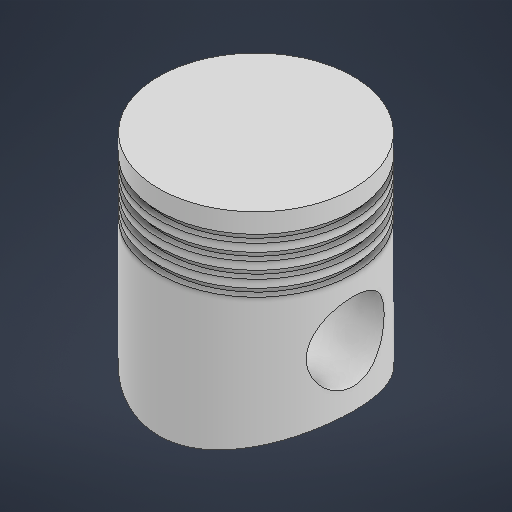
# Autodesk Inventor part: piston
Saved by Autodesk Inventor 2026.1 (Build 301233020, 233B)
## iProperties
Created: 2025-12-09
Part Number: piston
Material: Generic
Document SubType Name: Modeling
Designer: ender
Mass: 105.48 g
Surface Area: 374.417 cm^2
Volume: 105.48 cm^3
Density: 1 g/cm^3
Appearance: Default
Author: ender
Autodesk Inventor part; units mm, degrees
ref_plane "YZ Plane" through (0, 0, 0) normal (1, 0, 0) x (0, 1, 0)
ref_plane "XZ Plane" through (0, 0, 0) normal (0, 1, 0) x (-1, 0, 0)
ref_plane "XY Plane" through (0, 0, 0) normal (0, 0, 1) x (1, 0, 0)
sketch "Sketch1" plane through (0, 0, 0) normal (0, 0, 1) x (1, 0, 0)
  line L0 (0, 0) -> (31.75, 0)
  line L1 (31.75, 0) -> (31.75, -5.08)
  line L2 (31.75, -5.08) -> (0, -5.08)
  line L3 (0, -5.08) -> (0, 0)
  line L4 (31.75, -5.08) -> (26.67, -5.08)
  line L5 (26.67, -5.08) -> (26.67, -69.85)
  line L6 (26.67, -69.85) -> (31.75, -69.85)
  line L7 (31.75, -69.85) -> (31.75, -5.08)
  line L8 (0, 0) -> (0, 62.0882)
  line L9 (31.75, -6.35) -> (29.718, -6.35)
  line L10 (29.718, -6.35) -> (29.718, -8.89)
  line L11 (29.718, -8.89) -> (31.75, -8.89)
  line L12 (31.75, -8.89) -> (31.75, -6.35)
  line L13 (31.75, -11.43) -> (29.718, -11.43)
  line L14 (29.718, -11.43) -> (29.718, -13.97)
  line L15 (29.718, -13.97) -> (31.75, -13.97)
  line L16 (31.75, -13.97) -> (31.75, -11.43)
  line L17 (31.75, -16.51) -> (29.718, -16.51)
  line L18 (29.718, -16.51) -> (29.718, -19.05)
  line L19 (29.718, -19.05) -> (31.75, -19.05)
  line L20 (31.75, -19.05) -> (31.75, -16.51)
  line L21 (31.75, -21.59) -> (29.718, -21.59)
  line L22 (29.718, -21.59) -> (29.718, -24.13)
  line L23 (29.718, -24.13) -> (31.75, -24.13)
  line L24 (31.75, -24.13) -> (31.75, -21.59)
  line L25 (0, -96.2376) -> (0, 88.4758) projected
  dimension "d0" = 69.85
  dimension "d1" = 5.08
  dimension "d2" = 63.5
  dimension "d3" = 2.032
  dimension "d4" = 2.54
  dimension "d5" = 6.35
  dimension "d6" = 5.08
  dimension "d7" = 5.08
  dimension "d8" = 5.08
  constraints: 50 end point, 12 parallel, 6 horizontal, 6 perpendicular, 6 point on line, 4 equal length, 1 collinear, 1 vertical
  measures "d0" distance between parallel lines of L6 L0
  measures "d1" distance of L5.end L6.end
  measures "d2" diameter of L1 L8
  measures "d3" distance of L9.start L9.end
  measures "d4" distance of L9.end L10.end
  measures "d5" distance between parallel lines of L9 L0
  measures "d6" distance between parallel lines of L15 L11
  measures "d7" distance between parallel lines of L19 L15
  measures "d8" distance between parallel lines of L23 L19
revolve "Revolution1" add sketch "Sketch1" angle 360 about axis through (0, -10, 0) along (0, 1, 0) contours L0 L1 L2 L3 | L7 L9 L10 L11 L13 L14 L15 L17 L18 L19 L21 L22 L23 L6 L5 L2
sketch "Sketch2" plane through (0, -5.08, 0) normal (0, -1, 0) x (1, 0, 0)
  circle A0 centre (0, 0) radius 26.67 projected
  line L0 (20.9454, 16.51) -> (10.16, 16.51)
  line L1 (10.16, 16.51) -> (10.16, -16.51)
  line L2 (10.16, -16.51) -> (20.9454, -16.51)
  line L3 (-20.9454, 16.51) -> (-10.16, 16.51)
  line L4 (-10.16, 16.51) -> (-10.16, -16.51)
  line L5 (-10.16, -16.51) -> (-20.9454, -16.51)
  dimension "d10" = 33.02
  dimension "d11" = 20.32
  constraints: 12 end point, 4 equal length, 4 perpendicular, 4 point on circle, 2 horizontal
  measures "d10" distance between parallel lines of L5 L3
  measures "d11" distance between parallel lines of L4 L1
extrude "Extrusion1" add sketch "Sketch2" along normal blind 55.88 contours A0 L2 L1 L0 | L3 L4 L5 A0
sketch "Sketch3" plane through (-10.16, -5.08, 16.51) normal (1, 0, 0) x (0, 0, -1)
  circle A0 centre (16.51, -38.1) radius 12.7
  line L0 (48.26, 5.08) -> (-15.24, 5.08) projected
  point P0 (16.51, 5.08)
  dimension "d14" = 25.4
  dimension "d15" = 43.18
  constraints: 1 centre point, 1 vertical alignment
  measures "d14" diameter of A0
  measures "d15" distance from line of A0.centre L0
extrude "Extrusion2" cut sketch "Sketch3" along normal through all both and the other way through all
sketch "Sketch4" plane through (0, 0, 0) normal (1, 0, 0) x (0, 1, 0)
  line L0 (-69.85, -31.75) -> (-69.85, 31.75) projected
  arc A0 (-69.85, -31.75) -> (-69.85, 31.75) centre (-139.1203, 0) ccw
  point P0 (0, 0)
  dimension "d18" = 76.2
  constraints: 2 point on circle, 1 centre point
  measures "d18" radius of A0
extrude "Extrusion3" cut sketch "Sketch4" along normal through all both and the other way through all
body "Solid1"
